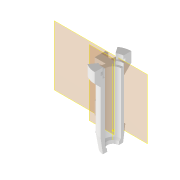
# Autodesk Inventor part: Voltera_Slide
Saved by Autodesk Inventor 2022 (Build 260153000, 153)
## iProperties
Created: 2022-08-22
Part Number: Voltera_Slide
Material: Generisch
Document SubType Name: Modeling
Designer: diederichbenedict
Density: 1 g/cm^3
Appearance: Vorgabe
Author: diederichbenedict
Autodesk Inventor part; units mm, degrees
ref_plane "YZ Plane" through (0, 0, 0) normal (1, 0, 0) x (0, 1, 0)
ref_plane "XZ Plane" through (0, 0, 0) normal (0, 1, 0) x (-1, 0, 0)
ref_plane "XY Plane" through (0, 0, 0) normal (0, 0, 1) x (1, 0, 0)
ref_plane "Arbeitsebene1" through (0, 0, 0) normal (0, 0, 1) x (1, 0, 0)
sketch "Skizze1" plane through (0, 0, 0) normal (0, 0, 1) x (1, 0, 0)
  line L0 (-4.8901, 59.5682) -> (-4.8901, -10.4318)
  line L1 (-22.7101, -0.4318) -> (-22.7101, 49.5682)
  line L2 (-16.7101, -0.4318) -> (-16.7101, 49.5682)
  circle A0 centre (-19.7101, 41.5682) radius 3 construction
  circle A1 centre (-19.7101, 7.5682) radius 3 construction
  line L3 (-25.7101, 47.5682) -> (-4.8901, 47.5682)
  line L4 (-4.8901, 47.5682) -> (-4.8901, 35.5682)
  line L5 (-4.8901, 35.5682) -> (-25.7101, 35.5682)
  line L6 (-25.7101, 35.5682) -> (-25.7101, 47.5682)
  line L7 (-4.8901, 13.5682) -> (-25.7101, 13.5682)
  line L8 (-25.7101, 13.5682) -> (-25.7101, 1.5682)
  line L9 (-25.7101, 1.5682) -> (-4.8901, 1.5682)
  line L10 (-4.8901, 1.5682) -> (-4.8901, 13.5682)
  circle A2 centre (-19.7101, 41.5682) radius 3.05
  circle A3 centre (-19.7101, 7.5682) radius 3.05
  line L11 (-4.8901, 35.5682) -> (-10.8901, 35.5682)
  line L12 (-10.8901, 35.5682) -> (-10.8901, 13.5682)
  line L13 (-10.8901, 13.5682) -> (-4.8901, 13.5682)
  line L14 (-4.8901, 13.5682) -> (-4.8901, 35.5682)
  point P0 (0, 0)
  point P1 (-4.8901, 1.5682)
  point P2 (-4.8901, 47.5682)
  point P3 (-16.7101, 41.0182)
  point P4 (-22.7101, 41.0182)
  point P5 (-22.7101, 42.1182)
  point P6 (-16.7101, 42.1182)
  dimension "d0" = 6
  dimension "d1" = 3
  dimension "d2" = 6
  dimension "d3" = 34
  dimension "d4" = 8
  dimension "d5" = 6
  dimension "d6" = 6
  dimension "d7" = 6
  dimension "d8" = 6
  dimension "d9" = 6
  dimension "d10" = 6
  dimension "d11" = 6.1
  dimension "d12" = 6.1
  dimension "d13" = 6
  constraints: 30 end point, 6 parallel, 4 centre point, 3 horizontal, 3 perpendicular, 3 point on line, 3 vertical, 2 coincident, 6 other
  measures "d0" diameter of A0
  measures "d1" distance from line of A0.centre L2
  measures "d2" diameter of A1
  measures "d3" distance of A0.centre A1.centre
  measures "d4" vertical distance of L2.end A0.centre
  measures "d5" distance from line of A0.centre L3
  measures "d6" distance from line of L5 A0.centre
  measures "d7" distance from line of L6 A0.centre
  measures "d8" distance from line of A1.centre L7
  measures "d9" distance from line of L9 A1.centre
  measures "d10" distance from line of L8 A1.centre
  measures "d11" diameter of A2
  measures "d12" diameter of A3
  measures "d13" distance between parallel lines of L14 L12
extrude "Extrusion1" add sketch "Skizze1" along normal blind 6 contours L0 L5 L2 A2 L3 | L0 L7 L12 L5 | L2 A2 L1 L3 | L0 L9 L2 A3 L7 | A2 L2 | L1 A2 L5 L6 L3 | L5 L1 A2 L2 | L1 A2 | L9 L1 A3 L2 | L2 A3 L1 L7 | L9 L8 L7 L1 A3
sketch "Skizze2" plane through (-25.7101, 47.5682, 0) normal (0, 1, 0) x (1, 0, 0)
  circle A0 centre (6, 3) radius 3 projected
  line L0 (0, 0) -> (0, 4)
  line L1 (0, 0) -> (4, 0) construction
  line L2 (0, 4) -> (2.6262, 4)
  line L3 (2.6262, 4) -> (3.698, 0)
  line L4 (0, 0) -> (14.82, 0) projected
  line L5 (9.3738, 4) -> (15.3738, 4)
  line L6 (15.3738, 4) -> (15.3738, 0)
  line L7 (15.3738, 0) -> (8.302, 0)
  line L8 (8.302, 0) -> (9.3738, 4)
  line L9 (30.8521, 0) -> (-5.142, 0) projected
  point P0 (25.7101, 0)
  point P1 (11.7707, 0)
  dimension "d16" = 4
  dimension "d17" = 90
  dimension "d18" = 15
  dimension "d19" = 15
  dimension "d22" = 6
  constraints: 16 end point, 4 perpendicular, 4 point on line, 2 tangent, 1 horizontal, 1 vertical
  measures "d16" distance of L0.start L0.end
  measures "d17" angle of L1 L0
  measures "d18" angle of L0 L3
  measures "d19" angle of L6 L8
  measures "d22" distance of L5.end L5.start
extrude "Extrusion2" add sketch "Skizze2" against normal up to surface (12 mm away) contours L3 L4 L0 L2 | L8 L5 L6 L7 L4
sketch "Skizze3" plane through (-25.7101, 13.5682, 0) normal (0, 1, 0) x (1, 0, 0)
  line L0 (20.82, 0) -> (15.3738, 0) projected
  line L1 (15.3738, 0) -> (15.3738, 4) projected
  line L2 (15.3738, 4) -> (9.3738, 4) projected
  line L3 (9.3738, 4) -> (8.302, 0) projected
  line L4 (8.302, 0) -> (3.698, 0) projected
  line L5 (3.698, 0) -> (2.6262, 4) projected
  line L6 (2.6262, 4) -> (0, 4) projected
  line L7 (0, 4) -> (0, -6) projected
  line L8 (20.82, -6) -> (0, -6) projected
  line L9 (20.82, 0) -> (20.82, -6) projected
  line L10 (0, 0) -> (0, -6) projected
  line L11 (0, 0) -> (3.698, 0)
  line L12 (8.302, 0) -> (15.3738, 0)
  point P0 (25.7101, 0)
  constraints: 4 end point, 1 collinear
extrude "Extrusion3" add sketch "Skizze3" against normal up to surface (12 mm away) contours L12 L3 L2 L1 | L11 L7 L6 L5
sketch "Skizze4" plane through (-22.012, 1.5682, 0) normal (0, -1, 0) x (1, 0, 0)
  line L0 (0, 0) -> (4.604, 0) projected
  line L1 (5.6758, -4) -> (4.604, 0) projected
  line L2 (11.6758, -4) -> (5.6758, -4) projected
  line L3 (11.6758, 0) -> (11.6758, -4) projected
  line L4 (11.6758, 0) -> (17.122, 0) projected
  line L5 (17.122, 0) -> (17.122, 6) projected
  line L6 (-3.698, 6) -> (17.122, 6) projected
  line L7 (-3.698, -4) -> (-3.698, 6) projected
  line L8 (-1.0718, -4) -> (-3.698, -4) projected
  line L9 (0, 0) -> (-1.0718, -4) projected
  circle A0 centre (17.122, 10) radius 7.325
  circle A1 centre (17.122, 10) radius 11.325
  line L10 (-3.698, 6) -> (11.1483, 19.6214)
  line L11 (-3.698, 6) -> (11.122, 6) projected
  line L12 (11.122, 6) -> (6.5269, 6)
  line L13 (17.122, 21.325) -> (17.122, 17.325)
  point P0 (8.0493, 16.7781)
  point P1 (10.9856, 6)
  point P2 (11.8064, 0)
  point P3 (17.122, 2.675)
  dimension "d27" = 14.65
  dimension "d28" = 10
  dimension "d29" = 4
  constraints: 6 end point, 3 point on circle, 1 centre point, 1 perpendicular, 1 point on line, 3 other
  measures "d28" distance from line of L0 A1.centre
extrude "Extrusion4" add sketch "Skizze4" against normal up to surface (46 mm away) contours A1 L10 L13 A0 L6 | L6 A0 L5 L4 A1
sketch "Skizze5" plane through (-4.8901, 47.5682, 6) normal (0, 1, 0) x (1, 0, 0)
  arc A0 (-6.1364, 0) -> (0, -11.325) centre (0, -4) ccw projected
  circle A1 centre (0, -4) radius 7.325
  point P0 (4.8901, 6)
  point P1 (0, -11.325)
  point P2 (-6.1364, 0)
  constraints: 1 centre point, 1 coincident, 1 concentric
extrude "Extrusion5" cut sketch "Skizze5" against normal through all
sketch "Skizze6" plane through (-4.8901, 1.5682, 0) normal (1, 0, 0) x (0, 0, -1)
  line L0 (-2.675, 46) -> (-2.675, 0) projected
  line L1 (0, 0) -> (-2.675, 0) projected
  line L2 (0, 0) -> (0, 46) projected
  line L3 (0, 46) -> (-2.675, 46) projected
  line L4 (0, 46) -> (4, 46) projected
  line L5 (0, 46) -> (7.644, 46) construction
  line L6 (6.75, 51.4052) -> (6.75, 55)
  line L7 (6.75, 55) -> (-0.5, 55)
  line L8 (-0.5, 55) -> (-0.5, 52)
  line L9 (-0.5, 52) -> (1.25, 52)
  line L10 (1.25, 52) -> (1.25, 49)
  line L11 (1.25, 49) -> (-0.5, 49)
  line L12 (-10, -12.8818) -> (-10, 66.3136) projected
  line L13 (-0.5, 49) -> (-0.5, 46)
  line L14 (4, 46) -> (-6, 46) projected
  line L15 (0, 34) -> (0, 46) projected
  line L16 (0, 38.848) -> (6.75, 45.598)
  line L17 (0, 38.848) -> (9.5459, 38.848) construction
  line L18 (6.75, 45.598) -> (6.75, 51.4052)
  line L19 (4, 46) -> (4, 34) projected
  line L20 (0, 38.848) -> (0, 46)
  line L21 (0, 46) -> (-0.5, 46)
  point P0 (0, -1.5682)
  dimension "d36" = 9.5
  dimension "d37" = 9.5
  dimension "d38" = 3
  dimension "d39" = 45
  dimension "d40" = 3
  dimension "d41" = 11.25
  dimension "d42" = 16.75
  dimension "d43" = 3
  constraints: 26 end point, 8 perpendicular, 2 horizontal, 2 point on line, 1 equal length, 1 parallel
  measures "d36" distance between parallel lines of L8 L12
  measures "d37" distance between parallel lines of L12 L13
  measures "d38" distance from line of L13.end L11
  measures "d39" angle of L17 L16
  measures "d40" distance between parallel lines of L9 L11
  measures "d41" distance between parallel lines of L12 L10
  measures "d42" distance between parallel lines of L12 L18
  measures "d43" distance between parallel lines of L7 L9
revolve "Umdrehung1" add sketch "Skizze6" angle 35 about axis through (-4.8901, 1.5682, 10) along (0, 1, 0) contours L13 L11 L10 L9 L8 L7 L6 L18 L16 L19 L4 L3 | L4 L19 L16 L2
ref_plane "Arbeitsebene2" through (-4.8901, 1.5682, 10) normal (0, 0, 1) x (1, 0, 0)
mirror "Spiegeln2" about plane through (-4.8901, 1.5682, 10) normal (0, 0, 1) of "Umdrehung1"
sketch "Skizze7" plane through (-4.8901, 1.5682, 10) normal (0, 0, 1) x (1, 0, 0)
  line L0 (0, 0) -> (0, 38.848) projected
  line L1 (0, 0) -> (-7.325, 0) projected
  line L2 (-11.325, 0) -> (-9.0727, 0) projected
  line L3 (0, 0) -> (0, -14)
  line L4 (0, -14) -> (-9.25, -14)
  line L5 (-9.25, -14) -> (-11.325, 0)
  line L6 (-11.4462, 0) -> (-9.0727, 0)
  line L7 (-5.4462, 0) -> (-11.4462, 0) projected
  line L8 (-5.6576, -11.2501) -> (-5.25, -14)
  line L9 (-9.25, -14) -> (-5.25, -14)
  line L10 (-7.325, 0) -> (-7.325, -9.8163)
  line L11 (-7.325, -9.8163) -> (-5.6576, -11.2501)
  point P0 (4.8901, -1.5682)
  point P1 (-10.5951, 0)
  dimension "d45" = 14
  dimension "d47" = 5.25
  constraints: 16 end point, 3 parallel, 2 vertical, 1 horizontal, 1 point on line
  measures "d45" distance of L0.start L3.end
  measures "d47" distance from line of L3 L8.end
revolve "Umdrehung2" add sketch "Skizze7" angle 180 mid plane about axis through (-4.8901, 1.5682, 10) along (0, -1, 0) contours L10 L11 L8 L4 L5 L2 L7
